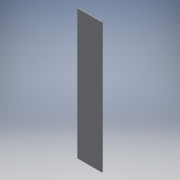
# Autodesk Inventor part: Top
Saved by Autodesk Inventor 2019 (Build 230136000, 136)
## iProperties
Created: 2018-09-21
Part Number: Top
Material: Generic
Document SubType Name: Modeling
Designer: user
Density: 1 g/cm^3
Appearance: Default
Author: user
Autodesk Inventor part; units mm, degrees
ref_plane "YZ Plane" through (0, 0, 0) normal (1, 0, 0) x (0, 1, 0)
ref_plane "XZ Plane" through (0, 0, 0) normal (0, 1, 0) x (-1, 0, 0)
ref_plane "XY Plane" through (0, 0, 0) normal (0, 0, 1) x (1, 0, 0)
sketch "Sketch1" plane through (0, 0, 0) normal (0, 0, 1) x (1, 0, 0)
  line L0 (-19.05, 0) -> (-19.05, 2438.4) projected
  line L1 (-19.05, 2438.4) -> (438.15, 2438.4)
  line L2 (438.15, 2438.4) -> (438.15, 0)
  line L3 (438.15, 0) -> (-19.05, 0)
  line L4 (-19.05, 0) -> (-19.05, 2438.4)
  point P0 (0, 0)
  point P1 (209.55, 0)
  dimension "d0" = 457.2
  constraints: 8 end point, 2 parallel, 1 horizontal, 1 horizontal alignment, 1 midpoint, 1 perpendicular
  measures "d0" distance of L2.end L3.end
extrude "Extrusion1" add sketch "Sketch1" along normal blind 19.05
body "Solid1"
